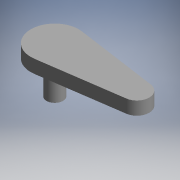
# Autodesk Inventor part: Servo_arm
Saved by Autodesk Inventor 2017 (Build 210142000, 142)
## iProperties
Part Number: Servo_arm
Material: Generic
Document SubType Name: Modeling
Designer: alex-
Appearance: Generic
Author: alex-
Autodesk Inventor part; units mm, degrees
ref_plane "YZ Plane" through (0, 0, 0) normal (1, 0, 0) x (0, 1, 0)
ref_plane "XZ Plane" through (0, 0, 0) normal (0, 1, 0) x (-1, 0, 0)
ref_plane "XY Plane" through (0, 0, 0) normal (0, 0, 1) x (1, 0, 0)
sketch "Sketch1" plane through (0, 0, 0) normal (0, 1, 0) x (-1, 0, 0)
  circle A0 centre (0, 0) radius 7.3033 construction
  circle A1 centre (-25, 0) radius 3.75 construction
  line L0 (-1.038, 7.2292) -> (-25.533, 3.7119)
  line L1 (-1.038, -7.2292) -> (-25.533, -3.7119)
  arc A2 (-1.038, -7.2292) -> (-1.038, 7.2292) centre (0, 0) ccw
  arc A3 (-25.533, 3.7119) -> (-25.533, -3.7119) centre (-25, 0) ccw
  dimension "d0" = 25
  dimension "d1" = 7.5
  constraints: 8 point on circle, 8 tangent, 4 centre point, 4 end point, 1 coincident
  measures "d0" distance of A1.centre point (0, 0)
  measures "d1" diameter of A1
extrude "Extrusion1" add sketch "Sketch1" along normal blind 4
sketch "Sketch2" plane through (0, 0, 0) normal (0, -1, 0) x (1, 0, 0)
  circle A0 centre (0, 0) radius 2.5
  dimension "d4" = 5
  constraints: 1 centre point, 1 coincident
  measures "d4" diameter of A0
extrude "Extrusion2" add sketch "Sketch2" along normal blind 10
body "Solid1"
